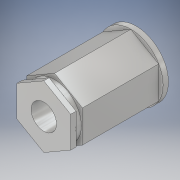
# Autodesk Inventor part: BaneBots-T40-6mm-Shaft-Adapter
Saved by Autodesk Inventor 2018 (Build 220112000, 112)
## iProperties
Created: 2017-12-20
Part Number: BaneBots-T40-6mm-Shaft-Adapter
Material: Generic
Document SubType Name: Modeling
Designer: jklei
Density: 1 g/cm^3
Appearance: Default
Author: jklei
Autodesk Inventor part; units mm, degrees
ref_plane "YZ Plane" through (0, 0, 0) normal (1, 0, 0) x (0, 1, 0)
ref_plane "XZ Plane" through (0, 0, 0) normal (0, 1, 0) x (-1, 0, 0)
ref_plane "XY Plane" through (0, 0, 0) normal (0, 0, 1) x (1, 0, 0)
sketch "Sketch3" plane through (0, 0, 0) normal (0, 0, 1) x (1, 0, 0)
  circle A0 centre (0, 0) radius 7.62
  dimension "d3" = 15.24
  constraints: 1 centre point, 1 coincident
  measures "d3" diameter of A0
extrude "Extrusion2" add sketch "Sketch3" along normal blind 1.27
sketch "Sketch4" plane through (0, 0, 1.27) normal (0, 0, 1) x (1, 0, 0)
  line L0 (0, 7.5994) -> (6.5813, 3.7997)
  line L1 (6.5813, 3.7997) -> (6.5813, -3.7997)
  line L2 (6.5813, -3.7997) -> (0, -7.5994)
  line L3 (0, -7.5994) -> (-6.5813, -3.7997)
  line L4 (-6.5813, -3.7997) -> (-6.5813, 3.7997)
  line L5 (-6.5813, 3.7997) -> (0, 7.5994)
  point P0 (0, 0)
  point P1 (0, 0)
  constraints: 12 end point, 1 coincident, 13 other
extrude "Extrusion3" add sketch "Sketch4" along normal blind 18.034
sketch "Sketch5" plane through (0, 0, 19.304) normal (0, 0, 1) x (1, 0, 0)
  circle A0 centre (0, 0) radius 6.35
  dimension "d8" = 12.7
  constraints: 1 centre point, 1 coincident
  measures "d8" diameter of A0
extrude "Extrusion4" add sketch "Sketch5" along normal blind 1.27
sketch "Sketch6" plane through (0, 0, 20.574) normal (0, 0, 1) x (1, 0, 0)
  circle A0 centre (0, 0) radius 6.35 projected
  line L0 (6.5813, 3.7997) -> (6.5813, -3.7997) projected
  line L1 (6.5813, -3.7997) -> (0, -7.5994) projected
  line L2 (0, -7.5994) -> (-6.5813, -3.7997) projected
  line L3 (-6.5813, -3.7997) -> (-6.5813, 3.7997) projected
  line L4 (-6.5813, 3.7997) -> (0, 7.5994) projected
  line L5 (0, 7.5994) -> (6.5813, 3.7997) projected
  circle A1 centre (0, 0) radius 7.62 projected
  line L6 (0, 7.5994) -> (6.5813, 3.7997) projected
  line L7 (6.35, 3.6662) -> (6.35, -3.6662)
  line L8 (6.35, -3.6662) -> (0, -7.3323)
  line L9 (0, -7.3323) -> (-6.35, -3.6662)
  line L10 (-6.35, -3.6662) -> (-6.35, 3.6662)
  line L11 (-6.35, 3.6662) -> (0, 7.3323)
  line L12 (0, 7.3323) -> (6.35, 3.6662)
  point P0 (3.175, 5.4993)
  constraints: 12 end point, 1 coincident, 1 midpoint, 15 other
extrude "Extrusion5" add sketch "Sketch6" along normal blind 1.27 contours A0 | L7 L8 A0 | A0 L12 L7 | A0 L11 L12 | L8 L9 A0 | A0 L10 L11 | L9 L10 A0
sketch "Sketch7" plane through (0, 0, 21.844) normal (0, 0, 1) x (1, 0, 0)
  circle A0 centre (0, 0) radius 3
  dimension "d13" = 6
  constraints: 1 centre point, 1 coincident
  measures "d13" diameter of A0
extrude "Extrusion6" cut sketch "Sketch7" against normal up to next
body "Solid2"
